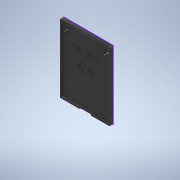
# Autodesk Inventor part: Top_latest(v3)
Saved by Autodesk Inventor 2022 (Build 260153000, 153)
## iProperties
Created: 2021-06-20
Part Number: Top_latest(v3)
Material: Generic
Document SubType Name: Modeling
Designer: micup
Density: 1 g/cm^3
Appearance: Glossy - Black
Author: micup
Autodesk Inventor part; units mm, degrees
ref_plane "YZ Plane" through (0, 0, 0) normal (1, 0, 0) x (0, 1, 0)
ref_plane "XZ Plane" through (0, 0, 0) normal (0, 1, 0) x (-1, 0, 0)
ref_plane "XY Plane" through (0, 0, 0) normal (0, 0, 1) x (1, 0, 0)
sketch "Sketch2" plane through (0, 0, 0) normal (0, 0, 1) x (1, 0, 0)
  line L0 (0, -0.4) -> (69, -0.4)
  line L1 (69, -0.4) -> (69, 94.6)
  line L2 (69, 94.6) -> (0, 94.6)
  line L3 (0, 94.6) -> (0, -0.4)
  line L4 (1.5, 1.1) -> (67.5, 1.1)
  line L5 (67.5, 1.1) -> (67.5, 93.1)
  line L6 (67.5, 93.1) -> (1.5, 93.1)
  line L7 (1.5, 93.1) -> (1.5, 1.1)
  line L8 (12, 82.6) -> (57, 82.6) construction
  line L9 (57, 82.6) -> (57, 12.6) construction
  line L10 (57, 12.6) -> (12, 12.6) construction
  line L11 (12, 12.6) -> (12, 82.6) construction
  line L12 (27, -0.4) -> (42, -0.4)
  line L13 (42, -0.4) -> (42, 1.1)
  line L14 (42, 1.1) -> (27, 1.1)
  line L15 (27, 1.1) -> (27, -0.4)
  line L16 (1, 0.6) -> (68, 0.6)
  line L17 (68, 0.6) -> (68, 93.6)
  line L18 (68, 93.6) -> (1, 93.6)
  line L19 (1, 93.6) -> (1, 0.6)
  line L20 (9, 0.6) -> (15, 0.6)
  line L21 (15, 0.6) -> (15, 0.2)
  line L22 (15, 0.2) -> (9, 0.2)
  line L23 (9, 0.2) -> (9, 0.6)
  line L24 (57, 0.2) -> (51, 0.2)
  line L25 (57, 0.6) -> (57, 0.2)
  line L26 (51, 0.2) -> (51, 0.6)
  line L27 (51, 0.6) -> (57, 0.6)
  line L28 (18, 93.6) -> (48, 93.6)
  line L29 (48, 93.6) -> (48, 94.1)
  line L30 (48, 94.1) -> (18, 94.1)
  line L31 (18, 94.1) -> (18, 93.6)
  line L32 (56.75, 4.1) -> (51.25, 4.1)
  line L33 (51, 3.85) -> (51, 2.6)
  line L34 (51, 2.6) -> (57, 2.6)
  line L35 (57, 2.6) -> (57, 3.85)
  line L36 (57, 2.6) -> (51, 2.6)
  line L37 (51, 2.6) -> (51, 2.45)
  line L38 (51.25, 2.2) -> (56.75, 2.2)
  line L39 (57, 2.45) -> (57, 2.6)
  arc A0 (57, 3.85) -> (56.75, 4.1) centre (56.75, 3.85) ccw
  arc A1 (51.25, 4.1) -> (51, 3.85) centre (51.25, 3.85) ccw
  arc A2 (51, 2.45) -> (51.25, 2.2) centre (51.25, 2.45) ccw
  arc A3 (56.75, 2.2) -> (57, 2.45) centre (56.75, 2.45) ccw
  line L40 (14.75, 4.1) -> (9.25, 4.1)
  line L41 (15, 2.6) -> (15, 3.85)
  arc A4 (15, 3.85) -> (14.75, 4.1) centre (14.75, 3.85) ccw
  arc A5 (14.75, 2.2) -> (15, 2.45) centre (14.75, 2.45) ccw
  line L42 (9, 2.6) -> (15, 2.6)
  line L43 (15, 2.45) -> (15, 2.6)
  line L44 (9.25, 2.2) -> (14.75, 2.2)
  arc A6 (9, 2.45) -> (9.25, 2.2) centre (9.25, 2.45) ccw
  line L45 (9, 3.85) -> (9, 2.6)
  arc A7 (9.25, 4.1) -> (9, 3.85) centre (9.25, 3.85) ccw
  line L46 (9, 2.6) -> (9, 2.45)
  line L47 (48, 91.6) -> (18, 91.6)
  line L48 (18, 91.6) -> (18, 90.35)
  line L49 (18.25, 90.1) -> (47.75, 90.1)
  line L50 (48, 90.35) -> (48, 91.6)
  line L51 (48, 91.6) -> (18, 91.6)
  line L52 (18, 91.6) -> (18, 91.75)
  line L53 (18.25, 92) -> (47.75, 92)
  line L54 (48, 91.75) -> (48, 91.6)
  arc A8 (18.25, 92) -> (18, 91.75) centre (18.25, 91.75) ccw
  arc A9 (18, 90.35) -> (18.25, 90.1) centre (18.25, 90.35) ccw
  arc A10 (47.75, 90.1) -> (48, 90.35) centre (47.75, 90.35) ccw
  arc A11 (48, 91.75) -> (47.75, 92) centre (47.75, 91.75) ccw
  circle A12 centre (6.5, 82.6) radius 3
  circle A13 centre (62.5, 82.6) radius 3
  point P0 (0, 0)
  point P1 (56.5, 81.5)
  point P2 (27, 1.1)
  point P3 (27, 1.1)
  point P4 (42, -0.4)
  point P5 (18, 92)
  dimension "d12" = 1.5
  dimension "d13" = 1.5
  dimension "d14" = 1.5
  dimension "d15" = 1.5
  dimension "d16" = 70
  dimension "d17" = 45
  dimension "d18" = 10.5
  dimension "d19" = 66
  dimension "d20" = 92
  dimension "d21" = 10.5
  dimension "d39" = 15
  dimension "d40" = 27
  dimension "d41" = 1
  dimension "d42" = 1
  dimension "d43" = 1
  dimension "d44" = 1
  dimension "d45" = 0.4
  dimension "d46" = 6
  dimension "d47" = 9
  dimension "d48" = 42
  dimension "d52" = 0.5
  dimension "d53" = 30
  dimension "d54" = 17
  dimension "d68" = 1.5
  dimension "d69" = 1.5
  dimension "d70" = 0.4
  dimension "d71" = 0.25
  dimension "d74" = 42
  dimension "d79" = 1.5
  dimension "d80" = 0.4
  dimension "d81" = 1.5
  dimension "d82" = 0.25
  dimension "d212" = 6
  dimension "d215" = 56
  dimension "d222" = 5
  constraints: 110 end point, 24 point on circle, 22 parallel, 16 tangent, 14 centre point, 14 horizontal, 11 perpendicular, 7 point on line, 6 equal radius, 1 collinear, 35 other
  measures "d12" distance between parallel lines of L2 L6
  measures "d13" distance between parallel lines of L0 L4
  measures "d14" distance between parallel lines of L1 L5
  measures "d15" distance between parallel lines of L3 L7
  measures "d16" distance between parallel lines of L10 L8
  measures "d17" distance between parallel lines of L9 L11
  measures "d18" distance between parallel lines of L7 L11
  measures "d19" distance between parallel lines of L5 L7
  measures "d20" distance between parallel lines of L4 L6
  measures "d21" distance between parallel lines of L6 L8
  measures "d39" distance between parallel lines of L13 L15
  measures "d40" distance between parallel lines of L3 L15
  measures "d41" distance between parallel lines of L2 L18
  measures "d42" distance between parallel lines of L1 L17
  measures "d43" distance between parallel lines of L3 L19
  measures "d44" distance between parallel lines of L0 L16
  measures "d45" distance between parallel lines of L16 L22
  measures "d46" distance between parallel lines of L21 L23
  measures "d47" distance between parallel lines of L23 L3
  measures "d48" distance of L22.start L24.start
  measures "d52" distance between parallel lines of L28 L30
  measures "d53" distance of L29.end L30.end
  measures "d54" distance from line of L19 L30.end
  measures "d68" distance between parallel lines of L4 L34
  measures "d69" distance between parallel lines of L34 L32
  measures "d70" distance between parallel lines of L34 L38
  measures "d71" radius of A0
  measures "d74" distance of L32.start L40.start
  measures "d79" distance between parallel lines of L6 L47
  measures "d80" distance between parallel lines of L53 L47
  measures "d81" distance between parallel lines of L49 L47
  measures "d82" radius of A8
  measures "d212" diameter of A12
  measures "d215" distance of A12.centre A13.centre
  measures "d222" distance from line of L7 A12.centre
extrude "Extrusion1" add sketch "Sketch2" along normal blind 1.5 contours L4 L7 L6 L5 | A0 L35 L34 L33 A1 L32 | L39 A3 L38 A2 L37 L34 | A4 L41 L42 L45 A7 L40 | L43 A5 L44 A6 L46 L42 | L50 A10 L49 A9 L48 L47 | L47 L52 A8 L53 A11 L54 | A12 | A13
extrude "Extrusion2" add sketch "Sketch2" along normal blind 4.5 contours L3 L2 L1 L0 L13 L16 L26 L24 L25 L17 L18 L29 L30 L31 L19 L23 L22 L21 L15 | L16 L19 L18 L17 L13 L4 L5 L6 L7 L15
extrude "Extrusion3" add sketch "Sketch2" along normal blind 4.5 contours L31 L30 L29 L18
extrude "Extrusion4" add sketch "Sketch2" along normal blind 4.5 contours L21 L22 L23 L16 | L16 L25 L24 L26
extrude "Extrusion7" add sketch "Sketch2" along normal blind 3 contours L15 L16 L13 L0 | L15 L4 L13 L16
sketch "Sketch3" plane through (0, 0, 1.5) normal (0, 0, 1) x (1, 0, 0)
  line L0 (0, 0) -> (63, 0)
  line L1 (63, 0) -> (63, 88)
  line L2 (63, 88) -> (0, 88)
  line L3 (0, 88) -> (0, 0)
  line L4 (1.5, 1.5) -> (61.5, 1.5)
  line L5 (61.5, 1.5) -> (61.5, 86.5)
  line L6 (61.5, 86.5) -> (1.5, 86.5)
  line L7 (1.5, 86.5) -> (1.5, 1.5)
  line L8 (9, 79) -> (54, 79) construction
  line L9 (54, 79) -> (54, 9) construction
  line L10 (54, 9) -> (9, 9) construction
  line L11 (9, 9) -> (9, 79) construction
  circle A0 centre (18.985, 69.431) radius 1.4
  circle A1 centre (44.015, 69.431) radius 1.4
  circle A2 centre (15.341, 31.556) radius 1.4
  circle A3 centre (47.659, 31.556) radius 1.4
  circle A4 centre (6.5, 81.5) radius 3
  circle A5 centre (56.5, 81.5) radius 3
  circle A6 centre (6.5, 6.5) radius 3
  circle A7 centre (56.5, 6.5) radius 3
  line L12 (25.5, 0) -> (37.5, 0)
  line L13 (37.5, 0) -> (37.5, 1.5)
  line L14 (37.5, 1.5) -> (25.5, 1.5)
  line L15 (25.5, 1.5) -> (25.5, 0)
  line L16 (1, 1) -> (62, 1)
  line L17 (62, 1) -> (62, 87)
  line L18 (62, 87) -> (1, 87)
  line L19 (1, 87) -> (1, 1)
  line L20 (7.5, 1) -> (13.5, 1)
  line L21 (13.5, 1) -> (13.5, 0.6)
  line L22 (13.5, 0.6) -> (7.5, 0.6)
  line L23 (7.5, 0.6) -> (7.5, 1)
  line L24 (55.5, 0.6) -> (49.5, 0.6)
  line L25 (55.5, 1) -> (55.5, 0.6)
  line L26 (49.5, 0.6) -> (49.5, 1)
  line L27 (49.5, 1) -> (55.5, 1)
  dimension "d101" = 1.5
  dimension "d102" = 1.5
  dimension "d103" = 1.5
  dimension "d104" = 1.5
  dimension "d105" = 70
  dimension "d106" = 45
  dimension "d107" = 7.5
  dimension "d108" = 60
  dimension "d109" = 85
  dimension "d110" = 7.5
  dimension "d111" = 2.8
  dimension "d112" = 2.8
  dimension "d113" = 2.8
  dimension "d114" = 2.8
  dimension "d115" = 6
  dimension "d116" = 6.341
  dimension "d117" = 6.341
  dimension "d118" = 9.985
  dimension "d119" = 9.985
  dimension "d120" = 22.556
  dimension "d121" = 22.556
  dimension "d122" = 9.569
  dimension "d123" = 9.569
  dimension "d124" = 5
  dimension "d125" = 5
  dimension "d126" = 50
  dimension "d127" = 75
  dimension "d128" = 12
  dimension "d129" = 25.5
  dimension "d130" = 1
  dimension "d131" = 1
  dimension "d132" = 1
  dimension "d133" = 1
  dimension "d134" = 0.4
  dimension "d135" = 6
  dimension "d136" = 7.5
  dimension "d137" = 42
  constraints: 56 end point, 12 parallel, 8 centre point, 8 horizontal, 6 perpendicular, 3 point on line, 1 vertical, 14 other
  measures "d101" distance between parallel lines of L2 L6
  measures "d102" distance between parallel lines of L0 L4
  measures "d103" distance between parallel lines of L1 L5
  measures "d104" distance between parallel lines of L3 L7
  measures "d105" distance between parallel lines of L10 L8
  measures "d106" distance between parallel lines of L9 L11
  measures "d107" distance between parallel lines of L7 L11
  measures "d108" distance between parallel lines of L5 L7
  measures "d109" distance between parallel lines of L4 L6
  measures "d110" distance between parallel lines of L6 L8
  measures "d111" diameter of A2
  measures "d112" diameter of A3
  measures "d113" diameter of A0
  measures "d114" diameter of A1
  measures "d115" diameter of A4
  measures "d116" distance from line of L11 A2.centre
  measures "d117" distance from line of L9 A3.centre
  measures "d118" distance from line of L11 A0.centre
  measures "d119" distance from line of L9 A1.centre
  measures "d120" distance from line of L10 A2.centre
  measures "d121" distance from line of L10 A3.centre
  measures "d122" distance from line of L8 A0.centre
  measures "d123" distance from line of L8 A1.centre
  measures "d124" distance from line of L6 A4.centre
  measures "d125" distance from line of L7 A4.centre
  measures "d126" distance of A4.centre A5.centre
  measures "d127" distance of A4.centre A6.centre
  measures "d128" distance between parallel lines of L13 L15
  measures "d129" distance between parallel lines of L3 L15
  measures "d130" distance between parallel lines of L2 L18
  measures "d131" distance between parallel lines of L1 L17
  measures "d132" distance between parallel lines of L3 L19
  measures "d133" distance between parallel lines of L0 L16
  measures "d134" distance between parallel lines of L16 L22
  measures "d135" distance between parallel lines of L21 L23
  measures "d136" distance between parallel lines of L23 L3
  measures "d137" distance of L22.start L25.end
extrude "Extrusion8" add sketch "Sketch2" along normal blind 3.5 contours L50 A10 L49 A9 L48 L47
sketch "Sketch4" plane through (18, 91.6, 1.5) normal (0, 1, 0) x (1, 0, 0)
  line L0 (30, -2) -> (0, -2) projected
  line L1 (30, 0) -> (30, -2) projected
  line L2 (0, -2) -> (30, -2)
  line L3 (30, -2) -> (30, -1.6)
  line L4 (30, -1.6) -> (0, -1.6)
  line L5 (0, -1.6) -> (0, -2)
  point P0 (-18, 1.5)
  dimension "d143" = 0.4
  constraints: 8 end point, 2 parallel, 1 horizontal, 1 perpendicular, 1 point on line
  measures "d143" distance between parallel lines of L0 L4
extrude "Extrusion9" add sketch "Sketch4" along normal blind 0.4
fillet "Fillet1" radius 0.5 1 edges at (33, 92, 3.5)
extrude "Extrusion10" add sketch "Sketch2" along normal blind 3.5 contours A0 L35 L34 L33 A1 L32 | A4 L41 L42 L45 A7 L40
sketch "Sketch5" plane through (51, 2.6, 1.5) normal (0, -1, 0) x (1, 0, 0)
  line L0 (-42, 0) -> (-42, 2) projected
  line L1 (-36, 0) -> (-36, 2) projected
  line L2 (-42, 2) -> (-36, 2)
  line L3 (-36, 2) -> (-36, 1.6)
  line L4 (-36, 1.6) -> (-42, 1.6)
  line L5 (-42, 1.6) -> (-42, 2)
  line L6 (6, 0) -> (6, 2) projected
  line L7 (0, 2) -> (6, 2)
  line L8 (6, 2) -> (6, 1.6)
  line L9 (6, 1.6) -> (0, 1.6)
  line L10 (0, 1.6) -> (0, 2)
  point P0 (-51, -1.5)
  dimension "d149" = 0.4
  dimension "d150" = 0.4
  constraints: 16 end point, 4 parallel, 2 horizontal, 2 perpendicular, 2 point on line
  measures "d149" distance between parallel lines of L2 L4
  measures "d150" distance between parallel lines of L7 L9
extrude "Extrusion11" add sketch "Sketch5" along normal blind 0.4
fillet "Fillet2" radius 0.5 2 edges at (12, 2.2, 3.5) (54, 2.2, 3.5)
fillet "Fillet3" radius 1 6 edges at (69, -0.4, 2.25) (0, -0.4, 2.25) (69, 94.6, 2.25) (0, 94.6, 2.25) (27, 0.35, 4.5) (42, 0.35, 4.5)
sketch "Sketch6" plane through (0, 0, 0) normal (0, 0, -1) x (-1, 0, 0)
  line L0 (-34.4999, 19.6) -> (-17.5294, 36.5706)
  line L1 (-17.5294, 36.5706) -> (-34.4999, 53.5411)
  line L2 (-34.4999, 53.5411) -> (-51.4705, 36.5706)
  line L3 (-51.4705, 36.5706) -> (-34.4999, 19.6)
  line L4 (-69, 0.6) -> (-69, 93.6) projected
  line L5 (0, 93.6) -> (0, 0.6) projected
  line L6 (-1, -0.4) -> (-68, -0.4) projected
  line L7 (-34.4999, 53.5411) -> (-40.2706, 59.3118) construction
  line L8 (-51.4705, 36.5706) -> (-60.7717, 45.8717) construction
  line L9 (-17.5294, 36.5706) -> (-5.1834, 24.2246) construction
  line L10 (-34.4999, 19.6) -> (-23.1281, 8.2281) construction
  line L11 (-36.692, 54.8846) -> (-39.1668, 57.3595)
  line L12 (-39.1668, 57.3595) -> (-40.5811, 55.9453)
  line L13 (-40.5811, 55.9453) -> (-38.1062, 53.4704)
  line L14 (-38.1062, 53.4704) -> (-36.692, 54.8846)
  line L15 (-41.0053, 55.521) -> (-42.4195, 54.1068)
  line L16 (-42.4195, 54.1068) -> (-39.9447, 51.6319)
  line L17 (-38.5304, 53.0462) -> (-41.0053, 55.521)
  line L18 (-39.9447, 51.6319) -> (-38.5304, 53.0462)
  line L19 (-42.8438, 53.6825) -> (-44.258, 52.2683)
  line L20 (-44.258, 52.2683) -> (-41.7831, 49.7935)
  line L21 (-40.3689, 51.2077) -> (-42.8438, 53.6825)
  line L22 (-41.7831, 49.7935) -> (-40.3689, 51.2077)
  line L23 (-44.6823, 51.8441) -> (-46.0965, 50.4299)
  line L24 (-46.0965, 50.4299) -> (-43.6216, 47.955)
  line L25 (-42.2074, 49.3692) -> (-44.6823, 51.8441)
  line L26 (-43.6216, 47.955) -> (-42.2074, 49.3692)
  line L27 (-46.5208, 50.0056) -> (-47.935, 48.5914)
  line L28 (-47.935, 48.5914) -> (-45.4601, 46.1165)
  line L29 (-44.0459, 47.5307) -> (-46.5208, 50.0056)
  line L30 (-45.4601, 46.1165) -> (-44.0459, 47.5307)
  line L31 (-48.3592, 48.1671) -> (-49.7734, 46.7529)
  line L32 (-49.7734, 46.7529) -> (-47.2986, 44.278)
  line L33 (-45.8844, 45.6922) -> (-48.3592, 48.1671)
  line L34 (-47.2986, 44.278) -> (-45.8844, 45.6922)
  line L35 (-50.1977, 46.3286) -> (-51.6119, 44.9144)
  line L36 (-51.6119, 44.9144) -> (-49.137, 42.4395)
  line L37 (-47.7228, 43.8538) -> (-50.1977, 46.3286)
  line L38 (-49.137, 42.4395) -> (-47.7228, 43.8538)
  line L39 (-52.0362, 44.4902) -> (-53.4504, 43.0759)
  line L40 (-53.4504, 43.0759) -> (-50.9755, 40.6011)
  line L41 (-49.5613, 42.0153) -> (-52.0362, 44.4902)
  line L42 (-50.9755, 40.6011) -> (-49.5613, 42.0153)
  line L43 (-53.8747, 42.6517) -> (-55.2889, 41.2375)
  line L44 (-55.2889, 41.2375) -> (-52.814, 38.7626)
  line L45 (-51.3998, 40.1768) -> (-53.8747, 42.6517)
  line L46 (-52.814, 38.7626) -> (-51.3998, 40.1768)
  line L47 (-16.1859, 34.3785) -> (-17.6001, 32.9643)
  line L48 (-17.6001, 32.9643) -> (-15.1252, 30.4894)
  line L49 (-13.711, 31.9037) -> (-16.1859, 34.3785)
  line L50 (-15.1252, 30.4894) -> (-13.711, 31.9037)
  line L51 (-18.0243, 32.5401) -> (-19.4386, 31.1258)
  line L52 (-19.4386, 31.1258) -> (-16.9637, 28.651)
  line L53 (-15.5495, 30.0652) -> (-18.0243, 32.5401)
  line L54 (-16.9637, 28.651) -> (-15.5495, 30.0652)
  line L55 (-19.8628, 30.7016) -> (-21.277, 29.2874)
  line L56 (-21.277, 29.2874) -> (-18.8022, 26.8125)
  line L57 (-17.388, 28.2267) -> (-19.8628, 30.7016)
  line L58 (-18.8022, 26.8125) -> (-17.388, 28.2267)
  line L59 (-21.7013, 28.8631) -> (-23.1155, 27.4489)
  line L60 (-23.1155, 27.4489) -> (-20.6406, 24.974)
  line L61 (-19.2264, 26.3882) -> (-21.7013, 28.8631)
  line L62 (-20.6406, 24.974) -> (-19.2264, 26.3882)
  line L63 (-23.5398, 27.0246) -> (-24.954, 25.6104)
  line L64 (-24.954, 25.6104) -> (-22.4791, 23.1355)
  line L65 (-21.0649, 24.5497) -> (-23.5398, 27.0246)
  line L66 (-22.4791, 23.1355) -> (-21.0649, 24.5497)
  line L67 (-25.3783, 25.1861) -> (-26.7925, 23.7719)
  line L68 (-26.7925, 23.7719) -> (-24.3176, 21.2971)
  line L69 (-22.9034, 22.7113) -> (-25.3783, 25.1861)
  line L70 (-24.3176, 21.2971) -> (-22.9034, 22.7113)
  line L71 (-27.2167, 23.3477) -> (-28.631, 21.9335)
  line L72 (-28.631, 21.9335) -> (-26.1561, 19.4586)
  line L73 (-24.7419, 20.8728) -> (-27.2167, 23.3477)
  line L74 (-26.1561, 19.4586) -> (-24.7419, 20.8728)
  line L75 (-29.0552, 21.5092) -> (-30.4694, 20.095)
  line L76 (-30.4694, 20.095) -> (-27.9946, 17.6201)
  line L77 (-26.5803, 19.0343) -> (-29.0552, 21.5092)
  line L78 (-27.9946, 17.6201) -> (-26.5803, 19.0343)
  line L79 (-30.8937, 19.6707) -> (-32.3079, 18.2565)
  line L80 (-32.3079, 18.2565) -> (-29.833, 15.7816)
  line L81 (-28.4188, 17.1958) -> (-30.8937, 19.6707)
  line L82 (-29.833, 15.7816) -> (-28.4188, 17.1958)
  line L83 (-52.814, 34.3785) -> (-54.9353, 32.2572)
  line L84 (-54.9353, 32.2572) -> (-53.5211, 30.843)
  line L85 (-53.5211, 30.843) -> (-51.3998, 32.9643)
  line L86 (-51.3998, 32.9643) -> (-52.814, 34.3785)
  line L87 (-51.4705, 36.5706) -> (-60.4154, 27.6257) construction
  line L88 (-34.4999, 19.6) -> (-42.4195, 11.6804) construction
  line L89 (-50.9755, 32.5401) -> (-53.0968, 30.4187)
  line L90 (-53.0968, 30.4187) -> (-51.6826, 29.0045)
  line L91 (-51.6826, 29.0045) -> (-49.5613, 31.1258)
  line L92 (-49.5613, 31.1258) -> (-50.9755, 32.5401)
  line L93 (-49.137, 30.7016) -> (-51.2584, 28.5803)
  line L94 (-51.2584, 28.5803) -> (-49.8442, 27.166)
  line L95 (-49.8442, 27.166) -> (-47.7228, 29.2874)
  line L96 (-47.7228, 29.2874) -> (-49.137, 30.7016)
  line L97 (-47.2986, 28.8631) -> (-49.4199, 26.7418)
  line L98 (-49.4199, 26.7418) -> (-48.0057, 25.3276)
  line L99 (-48.0057, 25.3276) -> (-45.8844, 27.4489)
  line L100 (-45.8844, 27.4489) -> (-47.2986, 28.8631)
  line L101 (-45.4601, 27.0246) -> (-47.5814, 24.9033)
  line L102 (-47.5814, 24.9033) -> (-46.1672, 23.4891)
  line L103 (-46.1672, 23.4891) -> (-44.0459, 25.6104)
  line L104 (-44.0459, 25.6104) -> (-45.4601, 27.0246)
  line L105 (-43.6216, 25.1861) -> (-45.7429, 23.0648)
  line L106 (-45.7429, 23.0648) -> (-44.3287, 21.6506)
  line L107 (-44.3287, 21.6506) -> (-42.2074, 23.7719)
  line L108 (-42.2074, 23.7719) -> (-43.6216, 25.1861)
  line L109 (-41.7831, 23.3477) -> (-43.9045, 21.2263)
  line L110 (-43.9045, 21.2263) -> (-42.4902, 19.8121)
  line L111 (-42.4902, 19.8121) -> (-40.3689, 21.9335)
  line L112 (-40.3689, 21.9335) -> (-41.7831, 23.3477)
  line L113 (-39.9447, 21.5092) -> (-42.066, 19.3879)
  line L114 (-42.066, 19.3879) -> (-40.6518, 17.9737)
  line L115 (-40.6518, 17.9737) -> (-38.5304, 20.095)
  line L116 (-38.5304, 20.095) -> (-39.9447, 21.5092)
  line L117 (-38.1062, 19.6707) -> (-40.2275, 17.5494)
  line L118 (-40.2275, 17.5494) -> (-38.8133, 16.1352)
  line L119 (-38.8133, 16.1352) -> (-36.692, 18.2565)
  line L120 (-36.692, 18.2565) -> (-38.1062, 19.6707)
  line L121 (-30.1866, 57.0059) -> (-32.3079, 54.8846)
  line L122 (-32.3079, 54.8846) -> (-30.8937, 53.4704)
  line L123 (-30.8937, 53.4704) -> (-28.7724, 55.5917)
  line L124 (-28.7724, 55.5917) -> (-30.1866, 57.0059)
  line L125 (-28.3481, 55.1675) -> (-30.4694, 53.0462)
  line L126 (-30.4694, 53.0462) -> (-29.0552, 51.6319)
  line L127 (-29.0552, 51.6319) -> (-26.9339, 53.7533)
  line L128 (-26.9339, 53.7533) -> (-28.3481, 55.1675)
  line L129 (-26.5096, 53.329) -> (-28.631, 51.2077)
  line L130 (-28.631, 51.2077) -> (-27.2167, 49.7935)
  line L131 (-27.2167, 49.7935) -> (-25.0954, 51.9148)
  line L132 (-25.0954, 51.9148) -> (-26.5096, 53.329)
  line L133 (-24.6712, 51.4905) -> (-26.7925, 49.3692)
  line L134 (-26.7925, 49.3692) -> (-25.3783, 47.955)
  line L135 (-25.3783, 47.955) -> (-23.2569, 50.0763)
  line L136 (-23.2569, 50.0763) -> (-24.6712, 51.4905)
  line L137 (-22.8327, 49.652) -> (-24.954, 47.5307)
  line L138 (-24.954, 47.5307) -> (-23.5398, 46.1165)
  line L139 (-23.5398, 46.1165) -> (-21.4185, 48.2378)
  line L140 (-21.4185, 48.2378) -> (-22.8327, 49.652)
  line L141 (-20.9942, 47.8136) -> (-23.1155, 45.6922)
  line L142 (-23.1155, 45.6922) -> (-21.7013, 44.278)
  line L143 (-21.7013, 44.278) -> (-19.58, 46.3993)
  line L144 (-19.58, 46.3993) -> (-20.9942, 47.8136)
  line L145 (-19.1557, 45.9751) -> (-21.277, 43.8538)
  line L146 (-21.277, 43.8538) -> (-19.8628, 42.4395)
  line L147 (-19.8628, 42.4395) -> (-17.7415, 44.5609)
  line L148 (-17.7415, 44.5609) -> (-19.1557, 45.9751)
  line L149 (-17.3172, 44.1366) -> (-19.4386, 42.0153)
  line L150 (-19.4386, 42.0153) -> (-18.0243, 40.6011)
  line L151 (-18.0243, 40.6011) -> (-15.903, 42.7224)
  line L152 (-15.903, 42.7224) -> (-17.3172, 44.1366)
  line L153 (-15.4788, 42.2981) -> (-17.6001, 40.1768)
  line L154 (-17.6001, 40.1768) -> (-16.1859, 38.7626)
  line L155 (-16.1859, 38.7626) -> (-14.0646, 40.8839)
  line L156 (-14.0646, 40.8839) -> (-15.4788, 42.2981)
  line L157 (-51.4705, 36.5706) -> (-17.5294, 36.5706) construction
  line L158 (-34.4999, 19.6) -> (-34.4999, 53.5411) construction
  circle A0 centre (-34.4999, 36.5706) radius 8.5
  circle A1 centre (-34.4999, 36.5706) radius 6.75
  line L159 (-36.8288, 43.9309) -> (-31.9618, 41.3692)
  line L160 (-36.8288, 43.9309) -> (-37.5274, 42.6035)
  line L161 (-37.5274, 42.6035) -> (-32.6604, 40.0418)
  line L162 (-32.6604, 40.0418) -> (-31.9618, 41.3692)
  line L163 (-48.5, 13.9467) -> (-20.5, 13.9467) construction
  line L164 (-20.5, 13.9467) -> (-20.5, 3.7834) construction
  line L165 (-20.5, 3.7834) -> (-48.5, 3.7834) construction
  line L166 (-48.5, 3.7834) -> (-48.5, 13.9467) construction
  line L167 (-33.1284, 47.9999) -> (-37.4861, 44.5287)
  line L168 (-33.1284, 47.9999) -> (-31.9638, 47.0098)
  line L169 (-31.9638, 47.0098) -> (-36.3216, 43.5386)
  line L170 (-36.3216, 43.5386) -> (-37.4861, 44.5287)
  spline S0 degree 2 poles (-39.8536, 8.8601) (-39.8536, 8.0049) (-40.6, 6.6604) (-41.1685, 6.2995) knots 0 0 0 1 2 2 2
  spline S1 degree 2 poles (-41.1685, 6.2995) (-41.643, 5.993) (-42.7602, 5.8151) (-43.388, 5.8151) knots 0 0 0 1 2 2 2
  line L171 (-43.388, 5.8151) -> (-45.2961, 5.8151)
  line L172 (-45.2961, 5.8151) -> (-45.2961, 11.9151)
  line L173 (-45.2961, 11.9151) -> (-43.4078, 11.9151)
  spline S2 degree 2 poles (-43.4078, 11.9151) (-42.7652, 11.9151) (-41.643, 11.7519) (-41.1487, 11.4356) knots 0 0 0 1 2 2 2
  spline S3 degree 2 poles (-41.1487, 11.4356) (-40.5506, 11.05) (-39.8536, 9.745) (-39.8536, 8.8601) knots 0 0 0 1 2 2 2
  spline S4 degree 2 poles (-41.4255, 8.87) (-41.4255, 9.4731) (-41.8408, 10.3332) (-42.2659, 10.5754) knots 0 0 0 1 2 2 2
  spline S5 degree 2 poles (-42.2659, 10.5754) (-42.5773, 10.7435) (-43.2595, 10.7781) (-43.734, 10.7781) knots 0 0 0 1 2 2 2
  line L174 (-43.734, 10.7781) -> (-43.7637, 10.7781)
  line L175 (-43.7637, 10.7781) -> (-43.7637, 6.957)
  line L176 (-43.7637, 6.957) -> (-43.734, 6.957)
  spline S6 degree 2 poles (-43.734, 6.957) (-43.2199, 6.957) (-42.513, 6.9916) (-42.1917, 7.1942) knots 0 0 0 1 2 2 2
  spline S7 degree 2 poles (-42.1917, 7.1942) (-41.816, 7.4315) (-41.4255, 8.2669) (-41.4255, 8.87) knots 0 0 0 1 2 2 2
  spline S8 degree 2 poles (-36.3142, 5.6964) (-37.6884, 5.6964) (-39.2999, 7.3574) (-39.2999, 8.8601) knots 0 0 0 1 2 2 2
  spline S9 degree 2 poles (-39.2999, 8.8601) (-39.2999, 10.3085) (-37.6835, 12.0337) (-36.3092, 12.0337) knots 0 0 0 1 2 2 2
  spline S10 degree 2 poles (-36.3092, 12.0337) (-35.9484, 12.0337) (-35.3651, 11.9497) (-35.0981, 11.8805) knots 0 0 0 1 2 2 2
  spline S11 degree 2 poles (-35.0981, 11.8805) (-34.8905, 11.8162) (-34.4011, 11.6036) (-34.2479, 11.5245) knots 0 0 0 1 2 2 2
  line L177 (-34.2479, 11.5245) -> (-34.2479, 10.0712)
  line L178 (-34.2479, 10.0712) -> (-34.4011, 10.0712)
  spline S12 degree 2 poles (-34.4011, 10.0712) (-34.5148, 10.1701) (-34.851, 10.4469) (-35.0635, 10.5754) knots 0 0 0 1 2 2 2
  spline S13 degree 2 poles (-35.0635, 10.5754) (-35.2761, 10.7089) (-35.7853, 10.8918) (-36.067, 10.8918) knots 0 0 0 1 2 2 2
  spline S14 degree 2 poles (-36.067, 10.8918) (-36.3982, 10.8918) (-36.9469, 10.6842) (-37.199, 10.4222) knots 0 0 0 1 2 2 2
  spline S15 degree 2 poles (-37.199, 10.4222) (-37.4264, 10.1899) (-37.7181, 9.394) (-37.7181, 8.8552) knots 0 0 0 1 2 2 2
  spline S16 degree 2 poles (-37.7181, 8.8552) (-37.7181, 8.2867) (-37.4165, 7.5106) (-37.1694, 7.2733) knots 0 0 0 1 2 2 2
  spline S17 degree 2 poles (-37.1694, 7.2733) (-36.9321, 7.041) (-36.3488, 6.8383) (-36.0571, 6.8383) knots 0 0 0 1 2 2 2
  spline S18 degree 2 poles (-36.0571, 6.8383) (-35.7556, 6.8383) (-35.2069, 7.041) (-35.019, 7.1646) knots 0 0 0 1 2 2 2
  spline S19 degree 2 poles (-35.019, 7.1646) (-34.8114, 7.2882) (-34.5, 7.5501) (-34.3863, 7.654) knots 0 0 0 1 2 2 2
  line L179 (-34.3863, 7.654) -> (-34.2479, 7.654)
  line L180 (-34.2479, 7.654) -> (-34.2479, 6.2204)
  spline S20 degree 2 poles (-34.2479, 6.2204) (-34.416, 6.1413) (-34.8559, 5.9436) (-35.0932, 5.8744) knots 0 0 0 1 2 2 2
  spline S21 degree 2 poles (-35.0932, 5.8744) (-35.3799, 5.7854) (-35.8792, 5.6964) (-36.3142, 5.6964) knots 0 0 0 1 2 2 2
  line L181 (-34.0007, 5.8151) -> (-31.9394, 11.9151)
  line L182 (-31.9394, 11.9151) -> (-30.2686, 11.9151)
  line L183 (-30.2686, 11.9151) -> (-28.2072, 5.8151)
  line L184 (-28.2072, 5.8151) -> (-29.7841, 5.8151)
  line L185 (-29.7841, 5.8151) -> (-30.1647, 7.0608)
  line L186 (-30.1647, 7.0608) -> (-32.0827, 7.0608)
  line L187 (-32.0827, 7.0608) -> (-32.4683, 5.8151)
  line L188 (-32.4683, 5.8151) -> (-34.0007, 5.8151)
  line L189 (-30.5009, 8.1681) -> (-31.1237, 10.1849)
  line L190 (-31.1237, 10.1849) -> (-31.7515, 8.1681)
  line L191 (-31.7515, 8.1681) -> (-30.5009, 8.1681)
  line L192 (-27.5992, 5.8151) -> (-27.5992, 11.9151)
  line L193 (-27.5992, 11.9151) -> (-23.4765, 11.9151)
  line L194 (-23.4765, 11.9151) -> (-23.4765, 10.7534)
  line L195 (-23.4765, 10.7534) -> (-26.0767, 10.7534)
  line L196 (-26.0767, 10.7534) -> (-26.0767, 9.6807)
  line L197 (-26.0767, 9.6807) -> (-23.6792, 9.6807)
  line L198 (-23.6792, 9.6807) -> (-23.6792, 8.519)
  line L199 (-23.6792, 8.519) -> (-26.0767, 8.519)
  line L200 (-26.0767, 8.519) -> (-26.0767, 6.9767)
  line L201 (-26.0767, 6.9767) -> (-23.4765, 6.9767)
  line L202 (-23.4765, 6.9767) -> (-23.4765, 5.8151)
  line L203 (-23.4765, 5.8151) -> (-27.5992, 5.8151)
  point P0 (0, 0)
  point P1 (-35.5215, 43.2428)
  point P2 (-34.3992, 45.07)
  dimension "d184" = 17
  dimension "d185" = 13.5
  dimension "d155" = 24
  dimension "d156" = 24
  dimension "d157" = 17.5295
  dimension "d159" = 20
  dimension "d160" = 2.5
  dimension "d161" = 0.6
  dimension "d162" = 2
  dimension "d165" = 2.6
  dimension "d168" = 32.5
  dimension "d171" = 2.5
  dimension "d172" = 2.5
  dimension "d173" = 0.6
  dimension "d174" = 2
  dimension "d177" = 2.6
  dimension "d180" = 32
  dimension "d183" = 2.5
  dimension "d192" = 1.5
  dimension "d194" = 5.5
  dimension "d199" = 28
  dimension "d200" = 20.5
  dimension "d205" = 1.5
  constraints: 328 end point, 9 parallel, 8 collinear, 7 perpendicular, 1 coincident, 1 horizontal alignment, 1 midpoint, 280 other
  measures "d155" distance between parallel lines of L0 L2
  measures "d156" distance between parallel lines of L1 L3
  measures "d157" distance from line of L4 L2.end
  measures "d159" distance from line of L6 L0.start
  measures "d160" distance between parallel lines of L2 L14
  measures "d161" distance between parallel lines of L7 L11
  measures "d162" distance between parallel lines of L11 L13
  measures "d165" distance of L11.end L15.start
  measures "d168" distance of L11.end L47.start
  measures "d171" distance between parallel lines of L47 L0
  measures "d172" distance between parallel lines of L3 L86
  measures "d173" distance between parallel lines of L87 L83
  measures "d174" distance between parallel lines of L85 L83
  measures "d177" distance of L83.start L89.start
  measures "d180" distance of L83.start L121.start
  measures "d183" distance between parallel lines of L122 L1
  measures "d192" distance between parallel lines of L159 L161
  measures "d194" distance between parallel lines of L162 L160
  measures "d199" distance between parallel lines of L164 L166
  measures "d200" distance between parallel lines of L4 L166
  measures "d205" distance between parallel lines of L169 L167
extrude "Extrusion12" add sketch "Sketch6" along normal blind 0.5 contours S0 S1 L171 L172 L173 S2 S3 | S8 S9 S10 S11 L177 L178 S12 S13 S14 S15 S16 S17 S18 S19 L179 L180 S20 S21 | L181 L182 L183 L184 L185 L186 L187 L188 | L192 L193 L194 L195 L196 L197 L198 L199 L200 L201 L202 L203
extrude "Extrusion14" add sketch "Sketch6" along normal blind 0.9 contours L3 L2 L1 L0 | A1 L161 L162 L159 picked at (-36.2313, 33.9278)
extrude "Extrusion16" add sketch "Sketch6" along normal blind 0.5 contours L14 L13 L12 L11 | L17 L18 L16 L15 | L21 L22 L20 L19 | L25 L26 L24 L23 | L29 L30 L28 L27 | L33 L34 L32 L31 | L37 L38 L36 L35 | L41 L42 L40 L39 | L45 L46 L44 L43 | L49 L50 L48 L47 | L53 L54 L52 L51 | L57 L58 L56 L55 | L61 L62 L60 L59 | L65 L66 L64 L63 | L69 L70 L68 L67 | L73 L74 L72 L71 | L77 L78 L76 L75 | L81 L82 L80 L79 | L86 L85 L84 L83 | L92 L91 L90 L89 | L96 L95 L94 L93 | L100 L99 L98 L97 | L104 L103 L102 L101 | L108 L107 L106 L105 | L112 L111 L110 L109 | L116 L115 L114 L113 | L120 L119 L118 L117 | L124 L123 L122 L121 | L128 L127 L126 L125 | L132 L131 L130 L129 | L136 L135 L134 L133 | L140 L139 L138 L137 | L144 L143 L142 L141 | L148 L147 L146 L145 | L152 L151 L150 L149 | L156 L155 L154 L153
extrude "Extrusion18" add sketch "Sketch2" along normal blind 4.5 contours A12 | A13
sketch "Sketch7" plane through (6.5, 82.6, 4.5) normal (0, 0, 1) x (1, 0, 0)
  circle A0 centre (0, 0) radius 2.5
  circle A1 centre (56, 0) radius 2.5
  point P0 (-6.5, -82.6)
  dimension "d225" = 5
  dimension "d226" = 56
  dimension "d227" = 5
  constraints: 2 centre point
  measures "d225" diameter of A0
  measures "d226" distance of A1.centre A0.centre
  measures "d227" diameter of A1
hole "Hole1" at (62.5, 82.6, 4.5) direction (0, 0, -1) diameter 5 depth 4
hole "Hole2" at (6.5, 82.6, 4.5) direction (0, 0, -1) diameter 5 depth 4
sketch "Sketch8" plane through (0, 0, 1.5) normal (0, 0, 1) x (1, 0, 0)
  line L0 (12.5, 73.1) -> (56.5, 73.1) construction
  line L1 (56.5, 73.1) -> (56.5, 38.4254) construction
  line L2 (56.5, 38.4254) -> (12.5, 38.4254) construction
  line L3 (12.5, 38.4254) -> (12.5, 73.1) construction
  line L4 (1.5, 1.1) -> (1.5, 93.1) projected
  line L5 (67.5, 93.1) -> (67.5, 1.1) projected
  line L6 (1.5, 93.1) -> (67.5, 93.1) projected
  line L7 (21.3632, 71.5105) -> (19.2673, 65.4105)
  line L8 (19.2673, 65.4105) -> (17.6706, 65.4105)
  line L9 (17.6706, 65.4105) -> (15.5747, 71.5105)
  line L10 (15.5747, 71.5105) -> (17.1615, 71.5105)
  line L11 (17.1615, 71.5105) -> (18.4912, 67.3729)
  line L12 (18.4912, 67.3729) -> (19.816, 71.5105)
  line L13 (19.816, 71.5105) -> (21.3632, 71.5105)
  spline S0 degree 2 poles (26.2472, 67.2593) (26.2472, 66.8094) (25.916, 66.0729) (25.5947, 65.8158) knots 0 0 0 1 2 2 2
  spline S1 degree 2 poles (25.5947, 65.8158) (25.2734, 65.5588) (24.3984, 65.2819) (23.7706, 65.2819) knots 0 0 0 1 2 2 2
  spline S2 degree 2 poles (23.7706, 65.2819) (23.0588, 65.2819) (22.0405, 65.5192) (21.7192, 65.6675) knots 0 0 0 1 2 2 2
  line L14 (21.7192, 65.6675) -> (21.7192, 66.9923)
  line L15 (21.7192, 66.9923) -> (21.8675, 66.9923)
  spline S3 degree 2 poles (21.8675, 66.9923) (22.2036, 66.7798) (23.1082, 66.4634) (23.4839, 66.4634) knots 0 0 0 1 2 2 2
  spline S4 degree 2 poles (23.4839, 66.4634) (23.7064, 66.4634) (24.2254, 66.5425) (24.4034, 66.671) knots 0 0 0 1 2 2 2
  spline S5 degree 2 poles (24.4034, 66.671) (24.5418, 66.7748) (24.7098, 67.0764) (24.7098, 67.3482) knots 0 0 0 1 2 2 2
  spline S6 degree 2 poles (24.7098, 67.3482) (24.7098, 67.6201) (24.4726, 67.9118) (24.2748, 67.981) knots 0 0 0 1 2 2 2
  spline S7 degree 2 poles (24.2748, 67.981) (24.0771, 68.0502) (23.5284, 68.065) (23.3158, 68.065) knots 0 0 0 1 2 2 2
  line L16 (23.3158, 68.065) -> (23.0538, 68.065)
  line L17 (23.0538, 68.065) -> (23.0538, 69.1377)
  line L18 (23.0538, 69.1377) -> (23.2961, 69.1377)
  spline S8 degree 2 poles (23.2961, 69.1377) (23.5729, 69.1377) (24.0425, 69.1871) (24.2056, 69.2613) knots 0 0 0 1 2 2 2
  spline S9 degree 2 poles (24.2056, 69.2613) (24.3688, 69.3404) (24.5517, 69.6172) (24.5517, 69.8545) knots 0 0 0 1 2 2 2
  spline S10 degree 2 poles (24.5517, 69.8545) (24.5517, 70.0423) (24.3786, 70.2746) (24.2551, 70.3389) knots 0 0 0 1 2 2 2
  spline S11 degree 2 poles (24.2551, 70.3389) (24.1068, 70.4131) (23.7113, 70.4625) (23.5729, 70.4625) knots 0 0 0 1 2 2 2
  spline S12 degree 2 poles (23.5729, 70.4625) (23.3504, 70.4625) (22.8808, 70.3587) (22.6633, 70.2746) knots 0 0 0 1 2 2 2
  spline S13 degree 2 poles (22.6633, 70.2746) (22.4903, 70.2104) (22.1146, 70.0028) (22.0256, 69.9484) knots 0 0 0 1 2 2 2
  line L19 (22.0256, 69.9484) -> (21.8971, 69.9484)
  line L20 (21.8971, 69.9484) -> (21.8971, 71.2534)
  spline S14 degree 2 poles (21.8971, 71.2534) (22.2135, 71.3869) (23.2812, 71.639) (23.8398, 71.639) knots 0 0 0 1 2 2 2
  spline S15 degree 2 poles (23.8398, 71.639) (24.3836, 71.639) (25.1844, 71.4511) (25.4662, 71.2682) knots 0 0 0 1 2 2 2
  spline S16 degree 2 poles (25.4662, 71.2682) (25.7776, 71.0755) (26.089, 70.4823) (26.089, 70.1115) knots 0 0 0 1 2 2 2
  spline S17 degree 2 poles (26.089, 70.1115) (26.089, 69.5875) (25.4859, 68.8065) (24.9916, 68.6928) knots 0 0 0 1 2 2 2
  line L21 (24.9916, 68.6928) -> (24.9916, 68.6335)
  spline S18 degree 2 poles (24.9916, 68.6335) (25.2091, 68.6038) (25.6244, 68.4456) (25.8221, 68.2677) knots 0 0 0 1 2 2 2
  spline S19 degree 2 poles (25.8221, 68.2677) (26.005, 68.1095) (26.2472, 67.6053) (26.2472, 67.2593) knots 0 0 0 1 2 2 2
  line L22 (32.0506, 63.9967) -> (26.5784, 63.9967)
  line L23 (26.5784, 63.9967) -> (26.5784, 64.8222)
  line L24 (26.5784, 64.8222) -> (32.0506, 64.8222)
  line L25 (32.0506, 64.8222) -> (32.0506, 63.9967)
  line L26 (37.0878, 65.4105) -> (32.6043, 65.4105)
  line L27 (32.6043, 65.4105) -> (32.6043, 66.4041)
  spline S20 degree 2 poles (32.6043, 66.4041) (33.1727, 66.8588) (34.0823, 67.6597) (34.4234, 68.0205) knots 0 0 0 1 2 2 2
  spline S21 degree 2 poles (34.4234, 68.0205) (34.8732, 68.4901) (35.2736, 69.2069) (35.2736, 69.5826) knots 0 0 0 1 2 2 2
  spline S22 degree 2 poles (35.2736, 69.5826) (35.2736, 70.0077) (34.7645, 70.4625) (34.3097, 70.4625) knots 0 0 0 1 2 2 2
  spline S23 degree 2 poles (34.3097, 70.4625) (34.0774, 70.4625) (33.6621, 70.3488) (33.4496, 70.2598) knots 0 0 0 1 2 2 2
  spline S24 degree 2 poles (33.4496, 70.2598) (33.2419, 70.1659) (32.9453, 69.9682) (32.8712, 69.9187) knots 0 0 0 1 2 2 2
  line L28 (32.8712, 69.9187) -> (32.7526, 69.9187)
  line L29 (32.7526, 69.9187) -> (32.7526, 71.2485)
  spline S25 degree 2 poles (32.7526, 71.2485) (33.0096, 71.3721) (34.107, 71.6291) (34.6162, 71.6291) knots 0 0 0 1 2 2 2
  spline S26 degree 2 poles (34.6162, 71.6291) (35.7037, 71.6291) (36.8209, 70.6602) (36.8209, 69.7853) knots 0 0 0 1 2 2 2
  spline S27 degree 2 poles (36.8209, 69.7853) (36.8209, 69.2464) (36.3117, 68.2084) (35.7235, 67.6152) knots 0 0 0 1 2 2 2
  spline S28 degree 2 poles (35.7235, 67.6152) (35.3527, 67.2494) (34.6557, 66.6809) (34.5025, 66.5623) knots 0 0 0 1 2 2 2
  line L30 (34.5025, 66.5623) -> (37.0878, 66.5623)
  line L31 (37.0878, 66.5623) -> (37.0878, 65.4105)
  spline S29 degree 2 poles (42.3524, 68.4605) (42.3524, 67.6695) (42.1003, 66.4832) (41.8185, 66.0828) knots 0 0 0 1 2 2 2
  spline S30 degree 2 poles (41.8185, 66.0828) (41.5417, 65.6873) (40.647, 65.2819) (40.0043, 65.2819) knots 0 0 0 1 2 2 2
  spline S31 degree 2 poles (40.0043, 65.2819) (39.3568, 65.2819) (38.467, 65.6873) (38.1852, 66.0926) knots 0 0 0 1 2 2 2
  spline S32 degree 2 poles (38.1852, 66.0926) (37.9034, 66.493) (37.6513, 67.6695) (37.6513, 68.4605) knots 0 0 0 1 2 2 2
  spline S33 degree 2 poles (37.6513, 68.4605) (37.6513, 69.2712) (37.9034, 70.418) (38.1902, 70.8332) knots 0 0 0 1 2 2 2
  spline S34 degree 2 poles (38.1902, 70.8332) (38.4769, 71.2386) (39.3815, 71.634) (40.0043, 71.634) knots 0 0 0 1 2 2 2
  spline S35 degree 2 poles (40.0043, 71.634) (40.6618, 71.634) (41.5417, 71.2188) (41.8235, 70.8085) knots 0 0 0 1 2 2 2
  spline S36 degree 2 poles (41.8235, 70.8085) (42.1003, 70.4081) (42.3524, 69.2267) (42.3524, 68.4605) knots 0 0 0 1 2 2 2
  spline S37 degree 2 poles (40.815, 68.4605) (40.815, 69.5925) (40.4443, 70.507) (40.0043, 70.507) knots 0 0 0 1 2 2 2
  spline S38 degree 2 poles (40.0043, 70.507) (39.5644, 70.507) (39.1887, 69.5925) (39.1887, 68.4555) knots 0 0 0 1 2 2 2
  spline S39 degree 2 poles (39.1887, 68.4555) (39.1887, 67.3383) (39.5644, 66.409) (40.0043, 66.409) knots 0 0 0 1 2 2 2
  spline S40 degree 2 poles (40.0043, 66.409) (40.4393, 66.409) (40.815, 67.3383) (40.815, 68.4605) knots 0 0 0 1 2 2 2
  line L32 (47.7752, 65.4105) -> (43.2916, 65.4105)
  line L33 (43.2916, 65.4105) -> (43.2916, 66.4041)
  spline S41 degree 2 poles (43.2916, 66.4041) (43.8601, 66.8588) (44.7697, 67.6597) (45.1107, 68.0205) knots 0 0 0 1 2 2 2
  spline S42 degree 2 poles (45.1107, 68.0205) (45.5606, 68.4901) (45.961, 69.2069) (45.961, 69.5826) knots 0 0 0 1 2 2 2
  spline S43 degree 2 poles (45.961, 69.5826) (45.961, 70.0077) (45.4518, 70.4625) (44.997, 70.4625) knots 0 0 0 1 2 2 2
  spline S44 degree 2 poles (44.997, 70.4625) (44.7647, 70.4625) (44.3495, 70.3488) (44.1369, 70.2598) knots 0 0 0 1 2 2 2
  spline S45 degree 2 poles (44.1369, 70.2598) (43.9293, 70.1659) (43.6327, 69.9682) (43.5586, 69.9187) knots 0 0 0 1 2 2 2
  line L34 (43.5586, 69.9187) -> (43.4399, 69.9187)
  line L35 (43.4399, 69.9187) -> (43.4399, 71.2485)
  spline S46 degree 2 poles (43.4399, 71.2485) (43.697, 71.3721) (44.7944, 71.6291) (45.3035, 71.6291) knots 0 0 0 1 2 2 2
  spline S47 degree 2 poles (45.3035, 71.6291) (46.391, 71.6291) (47.5082, 70.6602) (47.5082, 69.7853) knots 0 0 0 1 2 2 2
  spline S48 degree 2 poles (47.5082, 69.7853) (47.5082, 69.2464) (46.9991, 68.2084) (46.4108, 67.6152) knots 0 0 0 1 2 2 2
  spline S49 degree 2 poles (46.4108, 67.6152) (46.0401, 67.2494) (45.3431, 66.6809) (45.1898, 66.5623) knots 0 0 0 1 2 2 2
  line L36 (45.1898, 66.5623) -> (47.7752, 66.5623)
  line L37 (47.7752, 66.5623) -> (47.7752, 65.4105)
  line L38 (52.847, 65.4105) -> (48.8182, 65.4105)
  line L39 (48.8182, 65.4105) -> (48.8182, 66.4733)
  line L40 (48.8182, 66.4733) -> (50.1034, 66.4733)
  line L41 (50.1034, 66.4733) -> (50.1034, 69.7012)
  line L42 (50.1034, 69.7012) -> (48.8182, 69.7012)
  line L43 (48.8182, 69.7012) -> (48.8182, 70.6948)
  spline S50 degree 2 poles (48.8182, 70.6948) (49.1, 70.6948) (49.6586, 70.769) (49.8266, 70.8481) knots 0 0 0 1 2 2 2
  spline S51 degree 2 poles (49.8266, 70.8481) (50.0194, 70.9469) (50.2369, 71.2781) (50.2567, 71.5253) knots 0 0 0 1 2 2 2
  line L44 (50.2567, 71.5253) -> (51.5914, 71.5253)
  line L45 (51.5914, 71.5253) -> (51.5914, 66.4733)
  line L46 (51.5914, 66.4733) -> (52.847, 66.4733)
  line L47 (52.847, 66.4733) -> (52.847, 65.4105)
  spline S52 degree 2 poles (29.1464, 48.3685) (29.1464, 47.5134) (28.4, 46.1688) (27.8315, 45.8079) knots 0 0 0 1 2 2 2
  spline S53 degree 2 poles (27.8315, 45.8079) (27.357, 45.5014) (26.2398, 45.3235) (25.612, 45.3235) knots 0 0 0 1 2 2 2
  line L48 (25.612, 45.3235) -> (23.7039, 45.3235)
  line L49 (23.7039, 45.3235) -> (23.7039, 51.4235)
  line L50 (23.7039, 51.4235) -> (25.5922, 51.4235)
  spline S54 degree 2 poles (25.5922, 51.4235) (26.2348, 51.4235) (27.357, 51.2604) (27.8513, 50.944) knots 0 0 0 1 2 2 2
  spline S55 degree 2 poles (27.8513, 50.944) (28.4494, 50.5584) (29.1464, 49.2534) (29.1464, 48.3685) knots 0 0 0 1 2 2 2
  spline S56 degree 2 poles (27.5745, 48.3784) (27.5745, 48.9815) (27.1592, 49.8416) (26.7341, 50.0839) knots 0 0 0 1 2 2 2
  spline S57 degree 2 poles (26.7341, 50.0839) (26.4227, 50.2519) (25.7405, 50.2865) (25.266, 50.2865) knots 0 0 0 1 2 2 2
  line L51 (25.266, 50.2865) -> (25.2363, 50.2865)
  line L52 (25.2363, 50.2865) -> (25.2363, 46.4654)
  line L53 (25.2363, 46.4654) -> (25.266, 46.4654)
  spline S58 degree 2 poles (25.266, 46.4654) (25.7801, 46.4654) (26.487, 46.5) (26.8083, 46.7027) knots 0 0 0 1 2 2 2
  spline S59 degree 2 poles (26.8083, 46.7027) (27.184, 46.9399) (27.5745, 47.7754) (27.5745, 48.3784) knots 0 0 0 1 2 2 2
  spline S60 degree 2 poles (32.6858, 45.2048) (31.3116, 45.2048) (29.7001, 46.8658) (29.7001, 48.3685) knots 0 0 0 1 2 2 2
  spline S61 degree 2 poles (29.7001, 48.3685) (29.7001, 49.8169) (31.3165, 51.5421) (32.6908, 51.5421) knots 0 0 0 1 2 2 2
  spline S62 degree 2 poles (32.6908, 51.5421) (33.0516, 51.5421) (33.6349, 51.4581) (33.9019, 51.3889) knots 0 0 0 1 2 2 2
  spline S63 degree 2 poles (33.9019, 51.3889) (34.1095, 51.3246) (34.5989, 51.1121) (34.7521, 51.033) knots 0 0 0 1 2 2 2
  line L54 (34.7521, 51.033) -> (34.7521, 49.5796)
  line L55 (34.7521, 49.5796) -> (34.5989, 49.5796)
  spline S64 degree 2 poles (34.5989, 49.5796) (34.4852, 49.6785) (34.149, 49.9553) (33.9365, 50.0839) knots 0 0 0 1 2 2 2
  spline S65 degree 2 poles (33.9365, 50.0839) (33.7239, 50.2173) (33.2147, 50.4002) (32.933, 50.4002) knots 0 0 0 1 2 2 2
  spline S66 degree 2 poles (32.933, 50.4002) (32.6018, 50.4002) (32.0531, 50.1926) (31.801, 49.9306) knots 0 0 0 1 2 2 2
  spline S67 degree 2 poles (31.801, 49.9306) (31.5736, 49.6983) (31.2819, 48.9024) (31.2819, 48.3636) knots 0 0 0 1 2 2 2
  spline S68 degree 2 poles (31.2819, 48.3636) (31.2819, 47.7951) (31.5835, 47.019) (31.8306, 46.7818) knots 0 0 0 1 2 2 2
  spline S69 degree 2 poles (31.8306, 46.7818) (32.0679, 46.5494) (32.6512, 46.3467) (32.9429, 46.3467) knots 0 0 0 1 2 2 2
  spline S70 degree 2 poles (32.9429, 46.3467) (33.2444, 46.3467) (33.7931, 46.5494) (33.981, 46.673) knots 0 0 0 1 2 2 2
  spline S71 degree 2 poles (33.981, 46.673) (34.1886, 46.7966) (34.5, 47.0586) (34.6137, 47.1624) knots 0 0 0 1 2 2 2
  line L56 (34.6137, 47.1624) -> (34.7521, 47.1624)
  line L57 (34.7521, 47.1624) -> (34.7521, 45.7288)
  spline S72 degree 2 poles (34.7521, 45.7288) (34.584, 45.6497) (34.1441, 45.452) (33.9068, 45.3828) knots 0 0 0 1 2 2 2
  spline S73 degree 2 poles (33.9068, 45.3828) (33.6201, 45.2938) (33.1208, 45.2048) (32.6858, 45.2048) knots 0 0 0 1 2 2 2
  line L58 (34.9993, 45.3235) -> (37.0606, 51.4235)
  line L59 (37.0606, 51.4235) -> (38.7314, 51.4235)
  line L60 (38.7314, 51.4235) -> (40.7928, 45.3235)
  line L61 (40.7928, 45.3235) -> (39.2159, 45.3235)
  line L62 (39.2159, 45.3235) -> (38.8353, 46.5692)
  line L63 (38.8353, 46.5692) -> (36.9173, 46.5692)
  line L64 (36.9173, 46.5692) -> (36.5317, 45.3235)
  line L65 (36.5317, 45.3235) -> (34.9993, 45.3235)
  line L66 (38.4991, 47.6765) -> (37.8763, 49.6933)
  line L67 (37.8763, 49.6933) -> (37.2485, 47.6765)
  line L68 (37.2485, 47.6765) -> (38.4991, 47.6765)
  line L69 (41.4008, 45.3235) -> (41.4008, 51.4235)
  line L70 (41.4008, 51.4235) -> (45.5235, 51.4235)
  line L71 (45.5235, 51.4235) -> (45.5235, 50.2618)
  line L72 (45.5235, 50.2618) -> (42.9233, 50.2618)
  line L73 (42.9233, 50.2618) -> (42.9233, 49.1891)
  line L74 (42.9233, 49.1891) -> (45.3208, 49.1891)
  line L75 (45.3208, 49.1891) -> (45.3208, 48.0275)
  line L76 (45.3208, 48.0275) -> (42.9233, 48.0275)
  line L77 (42.9233, 48.0275) -> (42.9233, 46.4852)
  line L78 (42.9233, 46.4852) -> (45.5235, 46.4852)
  line L79 (45.5235, 46.4852) -> (45.5235, 45.3235)
  line L80 (45.5235, 45.3235) -> (41.4008, 45.3235)
  point P0 (0, 0)
  dimension "d242" = 11
  dimension "d243" = 11
  dimension "d244" = 20
  constraints: 2 other
  measures "d242" distance between parallel lines of L4 L3
  measures "d243" distance from line of L5 L1.end
  measures "d244" distance between parallel lines of L6 L0
emboss "Emboss1" sketch "Sketch8" operation cut depth 1 direction (0, 0, -1)
body "Solid1"
